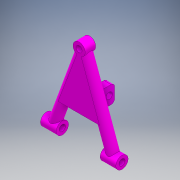
# Autodesk Inventor part: 下a臂
Saved by Autodesk Inventor 2019 (Build 230136000, 136)
## iProperties
Created: 2020-03-15
Part Number: 下a臂
Material: 一般
Document SubType Name: Modeling
Designer: 吳昇峻
Density: 1 g/cm^3
Appearance: 預設
Author: 吳昇峻
Autodesk Inventor part; units mm, degrees
sketch "草圖1" plane through (0, 0, 0) normal (0, 1, 0) x (-1, 0, 0)
  circle A0 centre (0, 0) radius 1.75
  circle A1 centre (0, 0) radius 3.5
  line L0 (0, 0) -> (-17.101, -46.9846) construction
  line L1 (0, 0) -> (50, 0) construction
  line L2 (0, 0) -> (17.101, -46.9846) construction
  line L3 (0, 0) -> (50, 0) construction
  line L4 (17.101, -46.9846) -> (-17.101, -46.9846) construction
  dimension "d0" = 3.5
  dimension "d1" = 7
  dimension "d5" = 50
  dimension "d6" = 110
  dimension "d7" = 50
  dimension "d8" = 70
  constraints: 10 end point, 2 centre point, 2 equal length, 2 horizontal, 1 coincident
  measures "d0" diameter of A0
  measures "d1" diameter of A1
  measures "d5" distance of L0.start L0.end
  measures "d6" angle of L0 L1
  measures "d7" distance of L0.start L2.end
  measures "d8" angle of L2 L3
extrude "擠出1" add sketch "草圖1" along normal mid plane 6
ref_plane "工作平面1" through (17.101, 0, -46.9846) normal (0, 0, 1) x (1, 0, 0)
ref_plane "工作平面2" through (17.101, 0, -46.9846) normal (1, 0, 0) x (0, 1, 0)
sketch "草圖4" plane through (17.101, 0, -46.9846) normal (1, 0, 0) x (0, 1, 0)
  circle A0 centre (0, 0) radius 1.75
  circle A1 centre (0, 0) radius 3.5
  point P0 (0, 46.9846)
  dimension "d22" = 3.5
  dimension "d23" = 7
  constraints: 2 centre point, 1 coincident
  measures "d22" diameter of A0
  measures "d23" diameter of A1
extrude "擠出3" add sketch "草圖4" along normal mid plane 9
mirror "鏡射1" about plane through (0, 0, 0) normal (1, 0, 0) of "擠出3"
sketch "草圖5" plane through (0, 0, 0) normal (0, 0, 1) x (1, 0, 0)
  circle A0 centre (0, 0) radius 3
  dimension "d26" = 6
  constraints: 1 centre point, 1 coincident
  measures "d26" diameter of A0
ref_plane "工作平面3" through (17.101, 0, -43.4846) normal (0, 0, 1) x (1, 0, 0)
sketch3d "3D 草圖1"
  line L0 (0, 0, 0) -> (17.101, 0, -46.9846)
sweep "掃掠1" add profiles "草圖5" path "3D 草圖1"
extrude "擠出4" cut sketch "草圖4" along normal mid plane 10 contours A0
mirror "鏡射2" about plane through (0, 0, 0) normal (1, 0, 0) of "掃掠1"
extrude "擠出7" cut sketch "草圖1" along normal through all both and the other way through all contours A0
ref_plane "工作平面4" through (-17.101, -1.75, -46.9846) normal (0, 0, 1) x (1, 0, 0)
extrude "擠出8" cut sketch "草圖4" along normal through all both and the other way through all contours A0
sketch "Sketch17" plane through (0, 0, 0) normal (0, 1, 0) x (-1, 0, 0)
  line L0 (0, 0) -> (0, -32) construction
  line L1 (0, 0) -> (-17.101, -46.9846) construction
  line L2 (0, -32) -> (-11.647, -32)
  line L3 (-11.647, -32) -> (0, 0)
  line L4 (0, 0) -> (12.093, -32)
  line L5 (12.093, -32) -> (0, -32)
  dimension "d76" = 32
  constraints: 10 end point, 2 collinear, 2 point on line, 1 horizontal, 1 vertical
  measures "d76" distance of L0.start L0.end
extrude "Extrusion13" add sketch "Sketch17" along normal mid plane 6
sketch "Sketch18" plane through (0, 3, 0) normal (0, 1, 0) x (1, 0, 0)
  line L0 (0, 0) -> (0, 24.5) construction
  line L1 (3.3, 29.5) -> (-3.3, 29.5) construction
  line L2 (-3.3, 29.5) -> (-3.3, 19.5) construction
  line L3 (-3.3, 19.5) -> (3.3, 19.5) construction
  line L4 (3.3, 19.5) -> (3.3, 29.5) construction
  line L5 (3.3, 29.5) -> (-3.3, 19.5) construction
  line L6 (-3.3, 29.5) -> (3.3, 19.5) construction
  line L7 (3.3, 29.5) -> (7.3, 29.5)
  line L8 (7.3, 29.5) -> (7.3, 19.5)
  line L9 (7.3, 19.5) -> (3.3, 19.5)
  line L10 (3.3, 19.5) -> (3.3, 29.5)
  line L11 (-3.3, 29.5) -> (-7.3, 29.5)
  line L12 (-7.3, 29.5) -> (-7.3, 19.5)
  line L13 (-7.3, 19.5) -> (-3.3, 19.5)
  line L14 (-3.3, 19.5) -> (-3.3, 29.5)
  dimension "d79" = 24.5
  dimension "d80" = 6.6
  dimension "d81" = 10
  dimension "d82" = 4
  dimension "d83" = 4
  constraints: 30 end point, 6 parallel, 3 horizontal, 3 perpendicular, 2 midpoint, 1 point on line, 1 vertical
  measures "d79" distance of L0.start L0.end
  measures "d80" distance of L3.end L2.end
  measures "d81" distance of L2.end L1.end
  measures "d82" distance of L8.end L9.end
  measures "d83" distance of L13.end L12.end
extrude "Extrusion14" add sketch "Sketch18" along normal blind 7
fillet "Fillet1" radius 2 4 edges at (-5.3, 10, -29.5) (-5.3, 10, -19.5) (5.3, 10, -19.5) (5.3, 10, -29.5)
sketch "Sketch19" plane through (-7.3, 3, -29.5) normal (-1, 0, 0) x (0, 0, 1)
  line L0 (10, 0) -> (0, 0) construction
  line L1 (5, 0) -> (5, 4) construction
  circle A0 centre (5, 4) radius 1.8
  point P0 (29.5, -3)
  dimension "d87" = 4
  dimension "d88" = 3.6
  constraints: 2 end point, 1 centre point, 1 coincident, 1 midpoint, 1 vertical
  measures "d87" distance of L1.start L1.end
  measures "d88" diameter of A0
extrude "Extrusion15" cut sketch "Sketch19" against normal through all
sketch "Sketch20" plane through (0, 3, 0) normal (0, 1, 0) x (1, 0, 0)
  arc A0 (-0.6186, 1.637) -> (0.5985, 1.6445) centre (0, 0) ccw projected
  circle A1 centre (0, 0) radius 1.75
  constraints: 1 centre point, 1 coincident, 1 concentric
extrude "Extrusion16" cut sketch "Sketch20" against normal blind 10
